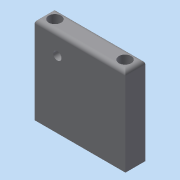
# Autodesk Inventor part: X smooth mount
Saved by Autodesk Inventor 2015 (Build 190159000, 159)
## iProperties
Created: 2016-09-08
Part Number: X smooth mount
Material: Generic
Document SubType Name: Modeling
Designer: Dustin
Density: 1 g/cm^3
Appearance: Default
Author: Dustin
Autodesk Inventor part; units mm, degrees
ref_plane "YZ Plane" through (0, 0, 0) normal (1, 0, 0) x (0, 1, 0)
ref_plane "XZ Plane" through (0, 0, 0) normal (0, 1, 0) x (-1, 0, 0)
ref_plane "XY Plane" through (0, 0, 0) normal (0, 0, 1) x (1, 0, 0)
sketch "Sketch1" plane through (0, 0, 0) normal (0, 0, 1) x (1, 0, 0)
  line L0 (0, 0) -> (44, 0)
  line L1 (44, 0) -> (44, 9.6635)
  line L2 (44, 9.6635) -> (0, 9.6635)
  line L3 (0, 9.6635) -> (0, 0)
  circle A0 centre (5, 4.8317) radius 3
  circle A1 centre (39, 4.8317) radius 3
  dimension "d0" = 6
  dimension "d1" = 6
  dimension "d2" = 34
  dimension "d3" = 44
  dimension "d4" = 5
  constraints: 8 end point, 2 centre point, 2 parallel, 1 horizontal, 1 perpendicular
  measures "d0" diameter of A0
  measures "d1" diameter of A1
  measures "d2" distance of A1.centre A0.centre
  measures "d3" distance of L1.end L2.end
  measures "d4" distance from line of L3 A0.centre
extrude "Extrusion1" add sketch "Sketch1" along normal blind 42.5
fillet "Fillet1" radius 2 4 edges at (22, 9.6635, 42.5) (0, 4.8317, 42.5) (22, 0, 42.5) (44, 4.8317, 42.5)
sketch "Sketch2" plane through (0, 9.6635, 0) normal (0, 1, 0) x (1, 0, 0)
  line L0 (44, 0) -> (0, 0) projected
  line L1 (0, 0) -> (0, -40.5) projected
  line L2 (5.9906, -42.5) -> (38.0094, -42.5) projected
  point P0 (11, -32.5)
  dimension "d17" = 10
  dimension "d18" = 11
  measures "d17" distance from line of L2 point (11, -32.5)
  measures "d18" distance from line of L1 point (11, -32.5)
hole "Hole1" at (11, 9.6635, 32.5) direction (0, -1, 0) diameter 4 depth 10 tip angle 118
body "Solid1"
